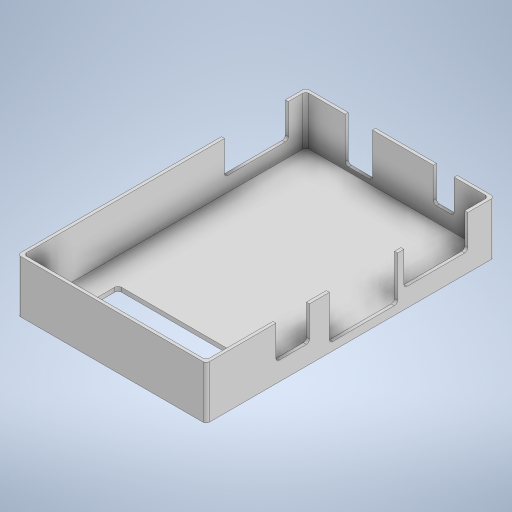
# Autodesk Inventor part: BoardCover
Saved by Autodesk Inventor 2023 (Build 270158000, 158)
## iProperties
Created: 2023-03-22
Part Number: BoardCover
Material: Generic
Document SubType Name: Modeling
Designer: User
Density: 1 g/cm^3
Appearance: Default
Author: User
Autodesk Inventor part; units mm, degrees
ref_plane "YZ Plane" through (0, 0, 0) normal (1, 0, 0) x (0, 1, 0)
ref_plane "XZ Plane" through (0, 0, 0) normal (0, 1, 0) x (-1, 0, 0)
ref_plane "XY Plane" through (0, 0, 0) normal (0, 0, 1) x (1, 0, 0)
sketch "Sketch1" plane through (0, 0, 0) normal (0, 1, 0) x (-1, 0, 0)
  line L0 (-45, 68.75) -> (45, 68.75)
  line L1 (45, 68.75) -> (45, -68.75)
  line L2 (45, -68.75) -> (-45, -68.75)
  line L3 (-45, -68.75) -> (-45, 68.75)
  line L4 (-45, 68.75) -> (45, -68.75) construction
  line L5 (45, 68.75) -> (-45, -68.75) construction
  point P0 (0, 0)
  dimension "d0" = 137.5
  dimension "d1" = 90
  constraints: 12 end point, 2 midpoint, 2 parallel, 1 horizontal, 1 perpendicular
  measures "d0" distance of L0.end L1.end
  measures "d1" distance of L1.end L2.end
extrude "Extrusion1" add sketch "Sketch1" along normal blind 25
sketch "Sketch2" plane through (0, 25, 0) normal (0, 1, 0) x (1, 0, 0)
  line L0 (43.55, -67.3) -> (-43.55, -67.3)
  line L1 (-43.55, -67.3) -> (-43.55, 67.3)
  line L2 (-43.55, 67.3) -> (43.55, 67.3)
  line L3 (43.55, 67.3) -> (43.55, -67.3)
  line L4 (43.55, -67.3) -> (-43.55, 67.3) construction
  line L5 (-43.55, -67.3) -> (43.55, 67.3) construction
  point P0 (0, 0)
  dimension "d4" = 134.6
  dimension "d5" = 87.1
  constraints: 12 end point, 2 midpoint, 2 parallel, 1 horizontal, 1 perpendicular
  measures "d4" distance of L0.end L1.end
  measures "d5" distance of L1.end L2.end
extrude "Extrusion2" cut sketch "Sketch2" against normal blind 23
sketch "Sketch4" plane through (0, 25, 0) normal (0, 1, 0) x (1, 0, 0)
  line L0 (-45, 68.75) -> (-45, -68.75) projected
  line L1 (-43.55, -67.3) -> (-43.55, 67.3) projected
  line L2 (-45, 59) -> (-43.55, 59)
  line L3 (-43.55, 59) -> (-43.55, 28.5)
  line L4 (-43.55, 28.5) -> (-45, 28.5)
  line L5 (-45, 28.5) -> (-45, 59)
  line L6 (41.75, -65.5) -> (-41.75, -65.5)
  line L7 (-41.75, -65.5) -> (-41.75, 65.5)
  line L8 (-41.75, 65.5) -> (41.75, 65.5)
  line L9 (41.75, 65.5) -> (41.75, -65.5)
  line L10 (41.75, -65.5) -> (-41.75, 65.5) construction
  line L11 (-41.75, -65.5) -> (41.75, 65.5) construction
  line L12 (-43.55, 67.3) -> (43.55, 67.3) projected
  line L13 (45, 68.75) -> (-45, 68.75) projected
  line L14 (17.25, 67.3) -> (27.25, 67.3)
  line L15 (27.25, 67.3) -> (27.25, 68.75)
  line L16 (27.25, 68.75) -> (17.25, 68.75)
  line L17 (17.25, 68.75) -> (17.25, 67.3)
  line L18 (43.55, 67.3) -> (43.55, -67.3) projected
  line L19 (45, -68.75) -> (45, 68.75) projected
  line L20 (43.55, 56) -> (45, 56)
  line L21 (45, 56) -> (45, 25.5)
  line L22 (45, 25.5) -> (43.55, 25.5)
  line L23 (43.55, 25.5) -> (43.55, 56)
  line L24 (43.55, -35.5) -> (45, -35.5)
  line L25 (45, -35.5) -> (45, -19.5)
  line L26 (45, -19.5) -> (43.55, -19.5)
  line L27 (43.55, -19.5) -> (43.55, -35.5)
  point P0 (0, 0)
  point P1 (45, 56)
  dimension "d10" = 30.5
  dimension "d11" = 131
  dimension "d12" = 83.5
  dimension "d13" = 6.5
  dimension "d16" = 10
  dimension "d17" = 14.5
  dimension "d18" = 30.5
  dimension "d19" = 9.5
  dimension "d20" = 30
  dimension "d21" = 16
  constraints: 44 end point, 10 parallel, 8 point on line, 5 horizontal, 5 perpendicular, 2 midpoint
  measures "d10" distance between parallel lines of L4 L2
  measures "d11" distance of L6.end L7.end
  measures "d12" distance of L7.end L8.end
  measures "d13" distance between parallel lines of L8 L2
  measures "d16" distance between parallel lines of L15 L17
  measures "d17" distance between parallel lines of L9 L15
  measures "d18" distance between parallel lines of L20 L22
  measures "d19" distance between parallel lines of L8 L20
  measures "d20" distance between parallel lines of L6 L24
  measures "d21" distance of L24.end L25.end
extrude "Extrusion4" cut sketch "Sketch4" against normal blind 16 contours L2 L1 L4 L0 | L13 L15 L12 L17 | L19 L22 L18 L20 | L19 L24 L18 L26
sketch "Sketch5" plane through (0, 25, 0) normal (0, 1, 0) x (1, 0, 0)
  line L0 (41.75, -65.5) -> (-41.75, -65.5)
  line L1 (-41.75, -65.5) -> (-41.75, 65.5)
  line L2 (-41.75, 65.5) -> (41.75, 65.5)
  line L3 (41.75, 65.5) -> (41.75, -65.5)
  line L4 (41.75, -65.5) -> (-41.75, 65.5) construction
  line L5 (-41.75, -65.5) -> (41.75, 65.5) construction
  line L6 (43.55, 25.5) -> (43.55, -19.5) projected
  line L7 (45, -19.5) -> (45, 25.5) projected
  line L8 (43.55, -10) -> (45, -10)
  line L9 (45, -10) -> (45, 22.5)
  line L10 (45, 22.5) -> (43.55, 22.5)
  line L11 (43.55, 22.5) -> (43.55, -10)
  line L12 (-43.55, 67.3) -> (43.55, 67.3) projected
  line L13 (45, 68.75) -> (-45, 68.75) projected
  line L14 (-11.75, 67.3) -> (-24.75, 67.3)
  line L15 (-24.75, 67.3) -> (-24.75, 68.75)
  line L16 (-24.75, 68.75) -> (-11.75, 68.75)
  line L17 (-11.75, 68.75) -> (-11.75, 67.3)
  point P0 (0, 0)
  point P1 (43.55, 22.5)
  dimension "d26" = 131
  dimension "d27" = 83.5
  dimension "d28" = 55.5
  dimension "d29" = 32.5
  dimension "d43" = 13
  dimension "d44" = 17
  constraints: 28 end point, 6 parallel, 4 point on line, 3 horizontal, 3 perpendicular, 2 midpoint
  measures "d26" distance of L0.end L1.end
  measures "d27" distance of L1.end L2.end
  measures "d28" distance between parallel lines of L0 L8
  measures "d29" distance between parallel lines of L8 L10
  measures "d43" distance between parallel lines of L15 L17
  measures "d44" distance between parallel lines of L1 L15
extrude "Extrusion5" cut sketch "Sketch5" against normal blind 21 contours L10 L7 L8 L6 | L15 L13 L17 L12
sketch "Sketch6" plane through (0, 2, 0) normal (0, 1, 0) x (1, 0, 0)
  line L0 (41.75, -67.5) -> (-41.75, -67.5)
  line L1 (-41.75, -67.5) -> (-41.75, 67.5)
  line L2 (-41.75, 67.5) -> (41.75, 67.5)
  line L3 (41.75, 67.5) -> (41.75, -67.5)
  line L4 (41.75, -67.5) -> (-41.75, 67.5) construction
  line L5 (-41.75, -67.5) -> (41.75, 67.5) construction
  line L6 (-31.25, -53.5) -> (31.75, -53.5)
  line L7 (31.75, -53.5) -> (31.75, -34.5)
  line L8 (31.75, -34.5) -> (-31.25, -34.5)
  line L9 (-31.25, -34.5) -> (-31.25, -53.5)
  point P0 (0, 0)
  dimension "d32" = 135
  dimension "d33" = 83.5
  dimension "d34" = 19
  dimension "d35" = 63
  dimension "d36" = 10
  dimension "d37" = 14
  constraints: 20 end point, 4 parallel, 2 horizontal, 2 midpoint, 2 perpendicular
  measures "d32" distance of L0.end L1.end
  measures "d33" distance of L1.end L2.end
  measures "d34" distance of L8.end L6.start
  measures "d35" distance of L7.end L8.end
  measures "d36" distance between parallel lines of L3 L7
  measures "d37" distance between parallel lines of L0 L6
extrude "Extrusion6" cut sketch "Sketch6" against normal through all contours L9 L8 L7 L6
fillet "Fillet1" radius 1.5 24 edges at (-43.55, 13.5, 67.3) (-43.55, 13.5, -67.3) (43.55, 13.5, -67.3) (43.55, 13.5, 67.3) (-31.25, 1, 34.5) (-31.25, 1, 53.5) (31.75, 1, 53.5) (31.75, 1, 34.5) (-44.275, 9, -28.5) (-44.275, 9, -59) (44.275, 9, 35.5) (44.275, 9, 19.5) (44.275, 4, 10) (44.275, 4, -22.5) (44.275, 9, -25.5) (44.275, 9, -56) (17.25, 9, -68.025) (27.25, 9, -68.025) (-45, 12.5, -68.75) (-45, 12.5, 68.75) (45, 12.5, 68.75) (45, 12.5, -68.75) (-11.75, 4, -68.025) (-24.75, 4, -68.025)
body "Solid1"
